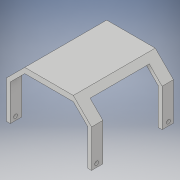
# Autodesk Inventor part: MotorProtector
Saved by Autodesk Inventor 2017 (Build 210142000, 142)
## iProperties
Created: 2017-11-28
Part Number: MotorProtector
Material: Generic
Document SubType Name: Modeling
Designer: User
Density: 1 g/cm^3
Appearance: Default
Author: User
Autodesk Inventor part; units mm, degrees
ref_plane "YZ Plane" through (0, 0, 0) normal (1, 0, 0) x (0, 1, 0)
ref_plane "XZ Plane" through (0, 0, 0) normal (0, 1, 0) x (-1, 0, 0)
ref_plane "XY Plane" through (0, 0, 0) normal (0, 0, 1) x (1, 0, 0)
sketch "Sketch1" plane through (0, 0, 0) normal (1, 0, 0) x (0, 1, 0)
  line L0 (0, 0) -> (46.736, 0)
  line L1 (46.736, 0) -> (46.736, -68.58)
  line L2 (46.736, -68.58) -> (0, -68.58)
  line L3 (0, -68.58) -> (0, 0)
  dimension "d0" = 46.736
  dimension "d1" = 68.58
  constraints: 8 end point, 2 parallel, 1 horizontal, 1 perpendicular
  measures "d0" distance of L1.end L2.end
  measures "d1" distance of L0.end L1.end
extrude "Extrusion1" add sketch "Sketch1" along normal blind 71.12
chamfer "Chamfer1" distance 15.24 angle 45 2 edges at (0, 46.736, -34.29) (71.12, 46.736, -34.29)
sketch "Sketch2" plane through (0, 0, 0) normal (0, 0, 1) x (1, 0, 0)
  line L0 (55.88, 46.736) -> (71.12, 31.496) projected
  line L1 (15.24, 46.736) -> (55.88, 46.736) projected
  line L2 (0, 31.496) -> (15.24, 46.736) projected
  line L3 (0, 0) -> (0, 31.496) projected
  line L4 (0, 0) -> (71.12, 0) projected
  line L5 (71.12, 31.496) -> (71.12, 0) projected
  line L6 (0, 0) -> (71.12, 0) projected
  line L7 (15.24, 42.2459) -> (55.88, 42.2459)
  line L8 (57.658, 0) -> (15.24, 0)
  line L9 (3.175, 0) -> (67.945, 0)
  line L10 (67.945, 0) -> (67.945, 30.1809)
  line L11 (3.175, 30.1809) -> (3.175, 0)
  line L12 (3.175, 30.1809) -> (15.24, 42.2459)
  line L13 (55.88, 42.2459) -> (67.945, 30.1809)
  dimension "d12" = 3.175
  dimension "d13" = 3.175
  dimension "d36" = 3.175
  dimension "d37" = 3.175
  dimension "d38" = 3.175
  dimension "d39" = 3.175
  constraints: 14 end point, 2 horizontal, 2 parallel, 2 point on line, 1 perpendicular
  measures "d12" distance between parallel lines of L5 L10
  measures "d13" distance between parallel lines of L3 L11
  measures "d36" distance from line of L2 L11.start
  measures "d37" distance from line of L2 L7.start
  measures "d38" distance from line of L0 L7.end
  measures "d39" distance from line of L0 L10.end
extrude "Extrusion2" cut sketch "Sketch2" against normal blind 127 contours L4 L11 L12 L7 L13 L10
sketch "Sketch3" plane through (71.12, 0, 0) normal (1, 0, 0) x (0, 0, -1)
  line L0 (0, 31.496) -> (68.58, 31.496) projected
  line L1 (0, 31.496) -> (0, 0) projected
  line L2 (0, 0) -> (68.58, 0) projected
  line L3 (68.58, 0) -> (68.58, 31.496) projected
  line L4 (4.2672, 3.175) -> (64.3128, 3.175)
  line L5 (64.3128, 3.175) -> (64.3128, 19.177)
  line L6 (64.3128, 19.177) -> (4.2672, 19.177)
  line L7 (4.2672, 19.177) -> (4.2672, 3.175)
  dimension "d16" = 60.0456
  dimension "d17" = 68.58
  dimension "d18" = 4.2672
  dimension "d19" = 16.002
  dimension "d20" = 31.496
  dimension "d21" = 3.175
  constraints: 8 end point, 2 parallel, 1 horizontal, 1 perpendicular
  measures "d16" distance of L4.start L4.end
  measures "d17" distance of L1.end L2.end
  measures "d18" distance between parallel lines of L1 L7
  measures "d19" distance of L4.end L5.end
  measures "d20" distance of L2.end L0.end
  measures "d21" distance between parallel lines of L2 L4
hole "Hole2" at (71.12, 3.175, -4.2672) at (71.12, 3.175, -64.3128) direction (-1, 0, 0) diameter 3.175 end through all
sketch "Sketch4" plane through (71.12, 0, 0) normal (1, 0, 0) x (0, 0, -1)
  circle A0 centre (4.2672, 3.175) radius 1.5875 projected
  circle A1 centre (64.3128, 3.175) radius 1.5875 projected
  line L0 (0, 31.496) -> (68.58, 31.496) projected
  line L1 (0, 31.496) -> (0, 0) projected
  line L2 (0, 0) -> (68.58, 0) projected
  line L3 (68.58, 0) -> (68.58, 31.496) projected
  line L4 (0, 46.736) -> (0, 31.496) projected
  line L5 (0, 31.496) -> (68.58, 31.496) projected
  line L6 (68.58, 31.496) -> (68.58, 46.736) projected
  line L7 (68.58, 46.736) -> (0, 46.736) projected
  line L8 (68.58, 0) -> (0, 0) projected
  line L9 (0, 42.2459) -> (68.58, 42.2459) projected
  line L10 (9.525, 0) -> (59.055, 0)
  line L11 (59.055, 0) -> (59.055, 42.2459)
  line L12 (59.055, 42.2459) -> (9.525, 42.2459)
  line L13 (9.525, 42.2459) -> (9.525, 0)
  dimension "d40" = 42.2459
  dimension "d41" = 68.58
  dimension "d42" = 49.53
  dimension "d43" = 9.525
  constraints: 8 end point, 2 parallel, 2 point on line, 1 horizontal, 1 perpendicular
  measures "d40" distance of L10.end L11.end
  measures "d41" distance of L6.end L4.start
  measures "d42" distance of L11.end L12.end
  measures "d43" distance between parallel lines of L1 L13
extrude "Extrusion3" cut sketch "Sketch4" against normal blind 127 contours L13 L9 L11 L0 | L0 L11 L2 L13
equation "\"d18\" = -0.5 * d16 + 0.5 * d17"
equation "\"d43\" = -0.5 * d42 + 0.5 * d41"
body "Solid1"
